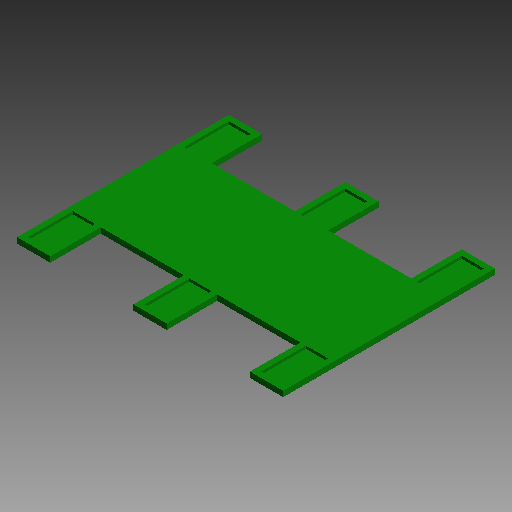
# Autodesk Inventor part: Body_bottom-01
Saved by Autodesk Inventor 2017 (Build 210142000, 142)
## iProperties
Part Number: Body_bottom-01
Material: Generic
Document SubType Name: Modeling
Designer: alex-
Appearance: Dark Green
b_mat_thickness: 0,500 cm
b_core_width: 10,000 cm
b_leg_space: 7,500 cm
Author: alex-
Autodesk Inventor part; units mm, degrees
ref_plane "YZ Plane" through (0, 0, 0) normal (1, 0, 0) x (0, 1, 0)
ref_plane "XZ Plane" through (0, 0, 0) normal (0, 1, 0) x (-1, 0, 0)
ref_plane "XY Plane" through (0, 0, 0) normal (0, 0, 1) x (1, 0, 0)
sketch "Sketch1" plane through (0, 0, 0) normal (0, 1, 0) x (-1, 0, 0)
  line L0 (120, 95.5) -> (90, 95.5)
  line L1 (120, -95.5) -> (90, -95.5)
  line L2 (120, 95.5) -> (120, -95.5)
  line L3 (90, 95.5) -> (90, 50)
  line L4 (90, -50) -> (90, -95.5)
  line L5 (90, 50) -> (15, 50)
  line L6 (90, -50) -> (15, -50)
  line L7 (15, 50) -> (15, 95.5)
  line L8 (15, -50) -> (15, -95.5)
  line L9 (15, 95.5) -> (-15, 95.5)
  line L10 (15, -95.5) -> (-15, -95.5)
  line L11 (-15, 95.5) -> (-15, 50)
  line L12 (-15, -50) -> (-15, -95.5)
  line L13 (-15, 50) -> (-90, 50)
  line L14 (-15, -50) -> (-90, -50)
  line L15 (-90, 50) -> (-90, 95.5)
  line L16 (-90, -50) -> (-90, -95.5)
  line L17 (-90, 95.5) -> (-120, 95.5)
  line L18 (-90, -95.5) -> (-120, -95.5)
  line L19 (-120, 95.5) -> (-120, -95.5)
  line L20 (120, 0) -> (-120, 0) construction
  line L21 (0, 95.5) -> (0, -95.5) construction
  point P0 (0, 0)
  point P1 (0, 0)
  dimension "d0" = 191
  dimension "b_servo_depth" = 30
  dimension "d3" = 75
  dimension "d4" = 45.5
  dimension "d5" = 100
  constraints: 44 end point, 16 equal length, 9 vertical, 8 horizontal, 6 horizontal alignment, 5 midpoint, 1 coincident, 1 parallel, 1 perpendicular
  measures "d0" distance of L0.start L1.start
  measures "b_servo_depth" distance of L0.start L0.end
  measures "d3" distance of L3.end L5.end
  measures "d4" distance of L0.end L3.end
  measures "d5" distance between parallel lines of L6 L5
extrude "Extrusion1" add sketch "Sketch1" along normal blind 5
sketch "Sketch2" plane through (0, 5, 0) normal (0, 1, 0) x (1, 0, 0)
  line L0 (-115, -90.5) -> (-95, -90.5)
  line L1 (-95, -90.5) -> (-95, -50)
  line L2 (-95, -50) -> (-115, -50)
  line L3 (-115, -50) -> (-115, -90.5)
  line L4 (-120, -95.5) -> (-90, -95.5) projected
  line L5 (-120, 95.5) -> (-120, -95.5) projected
  line L6 (-90, -95.5) -> (-90, -50) projected
  line L7 (-10, -90.5) -> (10, -90.5)
  line L8 (10, -90.5) -> (10, -50)
  line L9 (10, -50) -> (-10, -50)
  line L10 (-10, -50) -> (-10, -90.5)
  line L11 (95, -90.5) -> (115, -90.5)
  line L12 (115, -90.5) -> (115, -50)
  line L13 (115, -50) -> (95, -50)
  line L14 (95, -50) -> (95, -90.5)
  line L15 (-15, -50) -> (-15, -95.5) projected
  line L16 (90, -50) -> (90, -95.5) projected
  line L17 (-115, 50) -> (-95, 50)
  line L18 (-95, 50) -> (-95, 90.5)
  line L19 (-95, 90.5) -> (-115, 90.5)
  line L20 (-115, 90.5) -> (-115, 50)
  line L21 (-10, 50) -> (10, 50)
  line L22 (10, 50) -> (10, 90.5)
  line L23 (10, 90.5) -> (-10, 90.5)
  line L24 (-10, 90.5) -> (-10, 50)
  line L25 (95, 50) -> (115, 50)
  line L26 (115, 50) -> (115, 90.5)
  line L27 (115, 90.5) -> (95, 90.5)
  line L28 (95, 90.5) -> (95, 50)
  line L29 (-90, 95.5) -> (-120, 95.5) projected
  line L30 (-90, 50) -> (-90, 95.5) projected
  line L31 (-15, 95.5) -> (-15, 50) projected
  line L32 (90, 95.5) -> (90, 50) projected
  point P0 (0, 0)
  point P1 (-105, 50)
  point P2 (0, 50)
  point P3 (105, 50)
  point P4 (105, 90.5)
  point P5 (0, 90.5)
  point P6 (-105, 90.5)
  dimension "d8" = 5
  dimension "d9" = 5
  dimension "d10" = 5
  dimension "d11" = 40.5
  dimension "d12" = 5
  dimension "d13" = 5
  dimension "d14" = 5
  dimension "d15" = 5
  dimension "d16" = 5
  dimension "d17" = 40.5
  dimension "d18" = 5
  dimension "d19" = 5
  constraints: 48 end point, 12 parallel, 8 horizontal alignment, 6 horizontal, 6 midpoint, 6 perpendicular, 4 collinear, 4 point on line
  measures "d8" distance between parallel lines of L0 L4
  measures "d9" distance between parallel lines of L3 L5
  measures "d10" distance between parallel lines of L6 L1
  measures "d11" distance between parallel lines of L0 L2
  measures "d12" distance between parallel lines of L10 L15
  measures "d13" distance between parallel lines of L16 L14
  measures "d14" distance between parallel lines of L20 L5
  measures "d15" distance between parallel lines of L19 L29
  measures "d16" distance between parallel lines of L18 L30
  measures "d17" distance between parallel lines of L17 L19
  measures "d18" distance between parallel lines of L24 L31
  measures "d19" distance between parallel lines of L32 L28
extrude "Extrusion2" cut sketch "Sketch2" against normal blind 2.5
equation "\"b_servo_depth\" = s_depth + 2 * b_mat_thickness"
equation "\"d3\" = b_leg_space"
equation "\"d4\" = s_width + b_mat_thickness"
equation "\"d5\" = b_core_width"
equation "\"d6\" = b_mat_thickness"
equation "\"d8\" = b_mat_thickness"
equation "\"d9\" = b_mat_thickness"
equation "\"d10\" = b_mat_thickness"
equation "\"d11\" = s_width"
equation "\"d12\" = b_mat_thickness"
equation "\"d13\" = b_mat_thickness"
equation "\"d14\" = b_mat_thickness"
equation "\"d15\" = b_mat_thickness"
equation "\"d16\" = b_mat_thickness"
equation "\"d17\" = s_width"
equation "\"d18\" = b_mat_thickness"
equation "\"d19\" = b_mat_thickness"
equation "\"d20\" = 0.5 * b_mat_thickness"
equation "\"b_mat_thickness\" = 5"
equation "\"b_core_width\" = 100"
equation "\"b_leg_space\" = 75"
equation "\"s_depth\" = 20"
equation "\"s_width\" = 40.5"
body "Solid1"
